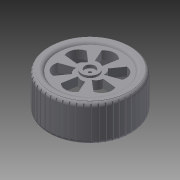
# Autodesk Inventor part: Wheels1
Saved by Autodesk Inventor 2015 (Build 190159000, 159)
## iProperties
Created: 2014-11-04
Part Number: Wheels1
Material: Generic
Document SubType Name: Modeling
Designer: ah14592
Density: 1 g/cm^3
Appearance: Default
Author: ah14592
Autodesk Inventor part; units mm, degrees
ref_plane "YZ Plane" through (0, 0, 0) normal (1, 0, 0) x (0, 1, 0)
ref_plane "XZ Plane" through (0, 0, 0) normal (0, 1, 0) x (-1, 0, 0)
ref_plane "XY Plane" through (0, 0, 0) normal (0, 0, 1) x (1, 0, 0)
sketch "Sketch1" plane through (0, 0, 0) normal (0, 1, 0) x (-1, 0, 0)
  line L0 (0, 0) -> (0, 48.3347) construction
  line L1 (-35, 49.2835) -> (-40, 49.2835)
  line L2 (-40, 49.2835) -> (-40, 14.2835)
  line L3 (-40, 14.2835) -> (-35, 14.2835)
  line L4 (-35, 14.2835) -> (-35, 49.2835)
  point P0 (0, 23.2008)
  dimension "d2" = 5
  dimension "d3" = 35
  dimension "d4" = 35
  constraints: 10 end point, 2 parallel, 2 vertical, 1 horizontal, 1 perpendicular, 1 point on line
  measures "d2" distance of L3.end L2.end
  measures "d3" distance of L2.end L1.end
  measures "d4" distance between parallel lines of L4 L0
revolve "Revolution1" add sketch "Sketch1" angle 360 about axis through (0, 0, 0) along (0, 0, 1)
fillet "Fillet1" radius 4 2 edges at (-40, 0, 49.2835) (-40, 0, 14.2835)
sketch "Sketch2" plane through (0, 0, 49.2835) normal (0, 0, 1) x (1, 0, 0)
  circle A0 centre (0, 0) radius 37.5
  dimension "d7" = 75
  constraints: 1 centre point, 1 coincident
  measures "d7" diameter of A0
extrude "Extrusion1" add sketch "Sketch2" against normal blind 10
fillet "Fillet2" radius 4 1 edges at (-35, 0, 39.2835)
sketch "Sketch3" plane through (0, 0, 49.2835) normal (0, 0, 1) x (1, 0, 0)
  circle A0 centre (0, 0) radius 40 construction
  line L0 (0, 40) -> (0, -40) construction
  line L1 (-40, 0) -> (40, 0) construction
  constraints: 4 end point, 4 point on circle, 1 perpendicular, 1 vertical
hole "Hole1" at (0, 0, 49.2835) direction (0, 0, -1) diameter 3 end through all counterbore diameter 10 counterbore depth 3
sketch "Sketch4" plane through (0, 0, 49.2835) normal (0, 0, 1) x (1, 0, 0)
  circle A0 centre (0, 0) radius 35 projected
  circle A1 centre (0, 0) radius 41 projected
  circle A2 centre (0, 0) radius 40 projected
  circle A3 centre (0, 0) radius 31 projected
  line L0 (-25.4682, 1.2657) -> (-12.5582, 0)
  line L1 (-18.5491, 15.2727) -> (-7.9173, 6.2441)
  arc A4 (-18.5491, 15.2727) -> (-25.4682, 1.2657) centre (-16.3717, 5.4847) ccw
  arc A5 (-7.9173, 6.2441) -> (-12.5582, 0) centre (-4.854, -0.8793) ccw
  circle A6 centre (0, 0) radius 1.5 construction
  line L2 (0, 0) -> (-39.644, 0) construction
  constraints: 6 end point, 4 point on circle, 2 centre point, 1 horizontal, 1 point on line
extrude "Extrusion2" cut sketch "Sketch4" against normal blind 10 contours A4 L1 A5 L0
sketch "Sketch5" plane through (0, 0, 49.2835) normal (0, 0, 1) x (1, 0, 0)
  circle A0 centre (0, 0) radius 31 projected
  circle A1 centre (0, 0) radius 35 projected
  circle A2 centre (0, 0) radius 1.5 projected
  circle A3 centre (0, 0) radius 31
  constraints: 1 centre point, 1 coincident, 1 concentric
extrude "Extrusion3" cut sketch "Sketch5" against normal blind 2 contours A0
fillet "Fillet3" radius 4 1 edges at (-31, 0, 49.2835)
pattern_circular "Circular Pattern1" count 6 over 360 about axis through (0, 0, -10) along (0, 0, 1) of "Extrusion2"
sketch "Sketch6" plane through (0, 0, 39.2835) normal (0, 0, -1) x (-1, 0, 0)
  circle A0 centre (0, 0) radius 31 construction
  line L0 (31, 0) -> (-31, 0) construction
  constraints: 2 end point, 2 point on circle, 1 horizontal
hole "Hole2" at (0, 0, 39.2835) direction (0, 0, 1) diameter 10 depth 2
sketch "Sketch7" plane through (0, 0, 49.2835) normal (0, 0, 1) x (1, 0, 0)
  circle A0 centre (0, 0) radius 40 projected
  line L0 (-40, 0) -> (-39, 0)
  line L1 (-39, 0) -> (-39, 1)
  line L2 (-39, 1) -> (-40, 1)
  line L3 (-40, 1) -> (-40, 0)
  dimension "d33" = 1
  dimension "d34" = 1
  constraints: 8 end point, 2 parallel, 1 horizontal, 1 horizontal alignment, 1 perpendicular, 1 other
  measures "d33" distance of L2.end L1.end
  measures "d34" distance of L1.end L0.end
extrude "Extrusion4" cut sketch "Sketch7" against normal up to next contours L3 L2 A0 | A0 L2 L1 L0 picked at (-39.3315, 0.5556)
pattern_circular "Circular Pattern2" count 50 over 360 about axis through (0, 0, -10) along (0, 0, 1) of "Extrusion4"
sketch "Sketch8" plane through (0, 0, 47.2835) normal (0, 0, 1) x (1, 0, 0)
  circle A0 centre (0, 0) radius 1.5 projected
  circle A1 centre (0, 0) radius 8
  circle A2 centre (0, 0) radius 5 projected
  circle A3 centre (0, 0) radius 5 projected
  circle A4 centre (0, 0) radius 1.5 projected
  dimension "d40" = 16
  constraints: 1 centre point, 1 coincident
  measures "d40" diameter of A1
extrude "Extrusion5" add sketch "Sketch8" along normal blind 2 contours A1
body "Solid1"
